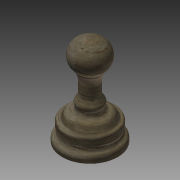
# Autodesk Inventor part: Pawn
Saved by Autodesk Inventor 2015 SP1 (Build 190203100, 203)
## iProperties
Created: 2015-06-07
Part Number: Pawn
Material: Generic
Document SubType Name: Modeling
Designer: Nathan
Density: 1 g/cm^3
Appearance: Driftwood
Author: Nathan
Autodesk Inventor part; units mm, degrees
ref_plane "YZ Plane" through (0, 0, 0) normal (1, 0, 0) x (0, 1, 0)
ref_plane "XZ Plane" through (0, 0, 0) normal (0, 1, 0) x (-1, 0, 0)
ref_plane "XY Plane" through (0, 0, 0) normal (0, 0, 1) x (1, 0, 0)
sketch "Sketch1" plane through (0, 0, 0) normal (0, 0, 1) x (1, 0, 0)
  arc A0 (7.1926, 34.8581) -> (0, 47) centre (1.69, 39.7998) ccw
  line L0 (0, 47) -> (0, 0)
  line L1 (0, 0) -> (14.846, 0)
  line L2 (4.4995, 27.8286) -> (4.4995, 22.431)
  arc A1 (12.9584, 6.4952) -> (13.7958, 3.4613) centre (14.831, 5.3796) ccw
  line L3 (13.2402, 9.7167) -> (13.2402, 7.5188)
  line L4 (14.846, 1.7013) -> (14.846, 0)
  arc A2 (12.9584, 6.4952) -> (13.2402, 7.5188) centre (11.2402, 7.5188) ccw
  arc A3 (14.846, 1.7013) -> (13.7958, 3.4613) centre (12.846, 1.7013) ccw
  arc A4 (7.1926, 34.8581) -> (4.4995, 27.8286) centre (15.02, 27.8286) ccw
  arc A5 (13.2402, 9.7167) -> (12.1426, 10.7119) centre (12.2402, 9.7167) ccw
  arc A6 (11.1978, 11.1758) -> (12.1426, 10.7119) centre (12.045, 11.7072) ccw
  arc A7 (4.4995, 22.431) -> (4.8051, 21.3684) centre (6.4995, 22.431) ccw
  arc A8 (6.0119, 17.5245) -> (8.1288, 14.1494) centre (8.019, 16.4319) ccw
  line L5 (4.8051, 21.3684) -> (5.9497, 19.5435)
  line L6 (9.9193, 13.2144) -> (11.1978, 11.1758)
  arc A9 (6.0119, 17.5245) -> (5.9497, 19.5435) centre (4.2554, 18.4808) ccw
  arc A10 (9.9193, 13.2144) -> (8.1288, 14.1494) centre (8.2249, 12.1517) ccw
  point P0 (4.4995, 32.9583)
  point P1 (14.846, 3.1999)
  point P2 (13.2402, 6.8697)
  point P3 (12.2402, 10.7167)
  point P4 (9.1475, 14.4448)
  point P5 (6.7214, 18.313)
  dimension "d11" = 2
  dimension "d13" = 1
  dimension "d14" = 1
  dimension "d15" = 2
  dimension "d16" = 2
  constraints: 28 point on circle, 17 tangent, 14 end point, 11 centre point, 5 point on line, 3 vertical, 2 equal radius, 1 horizontal
  measures "d11" radius of A2
  measures "d13" radius of A5
  measures "d14" radius of A6
  measures "d15" radius of A7
  measures "d16" radius of A9
revolve "Revolution1" add sketch "Sketch1" angle 360 about axis through (0, 47, 0) along (0, -1, 0)
body "Solid1"
